Parametric_HexGrid_Generator v1 (Autodesk Fusion 360 design; units mm, degrees)
Autodesk Fusion 360 part; units mm, degrees
note: some values were not read from the file. Chosen so that the rebuilt part matches the saved one: which bodies a step acts on; which face or edge a step refers to.
sketch "Sketch1" plane through (0, 0, 0) normal (0, 1, 0) x (1, 0, 0)
  line L0 (60, 20) -> (-60, 20)
  line L1 (-60, 20) -> (-60, -20)
  line L2 (-60, -20) -> (60, -20)
  line L3 (60, -20) -> (60, 20)
  line L4 (60, 20) -> (-60, -20) construction
  line L5 (-60, 20) -> (60, -20) construction
  line L6 (-57, -17) -> (57, -17)
  line L7 (57, -17) -> (57, 17)
  line L8 (57, 17) -> (-57, 17)
  line L9 (-57, 17) -> (-57, -17)
  line L10 (6, 3.4641) -> (0, 6.9282)
  line L11 (0, 6.9282) -> (-6, 3.4641)
  line L12 (-6, 3.4641) -> (-6, -3.4641)
  line L13 (-6, -3.4641) -> (0, -6.9282)
  line L14 (0, -6.9282) -> (6, -3.4641)
  line L15 (6, -3.4641) -> (6, 3.4641)
  line L16 (0, 0) -> (3, 5.1962) construction
  line L17 (0, 0) -> (6, 0) construction
  line L18 (120, 40) -> (-120, 40)
  line L19 (-120, 40) -> (-120, -40)
  line L20 (-120, -40) -> (120, -40)
  line L21 (120, -40) -> (120, 40)
  line L22 (120, 40) -> (-120, -40) construction
  line L23 (-120, 40) -> (120, -40) construction
  dimension "d6" = 120
  dimension "d7" = 40
  dimension "d9" = 6
  dimension "d27" = 240
  dimension "d28" = 80
  constraint horizontal L0
  constraint perpendicular L0 L1
  constraint parallel L0 L2
  constraint parallel L1 L3
  constraint coincident L4 L16.start
  constraint coincident L5 L16.start
  constraint coincident L16.start L17.start
  constraint vertical L15
  constraint midpoint L10 L16.end
  constraint midpoint L15 L17.end
  constraint horizontal L18
  constraint perpendicular L18 L19
  constraint parallel L18 L20
  constraint parallel L19 L21
  constraint coincident L22 L16.start
  constraint coincident L23 L16.start
  measures "d6" distance of L1.end L2.end
  measures "d7" distance of L0.end L1.end
  measures "d9" distance of L16.start L15
  measures "d27" distance of L19.end L20.end
  measures "d28" distance of L18.end L19.end
extrude "Extrude1" add sketch "Sketch1" along normal blind 5 contours L6 L7 L8 L9 | L10 L11 L12 L13 L14 L15 makes body 1
extrude "Extrude2" cut sketch "Sketch1" along normal blind 5 contours L10 L11 L12 L13 L14 L15 bodies 1
fillet "Fillet1" radius 1 6 edges at (6, 2.5, 3.4641) (6, 2.5, -3.4641) (0, 2.5, -6.9282) (-6, 2.5, -3.4641) (-6, 2.5, 3.4641) (0, 2.5, 6.9282) on bodies 1
extrude "Extrude3" add sketch "Sketch1" along normal blind 5 contours L0 L1 L2 L3 | L18 L19 L20 L21 bodies 1
extrude "Extrude4" add sketch "Sketch1" along normal blind 5 separate body contours L0 L1 L2 L3 makes body 2
pattern_linear "R-Pattern1" count 11 spacing 15 along (1, 0, 0) both ways count 4 spacing 15 along (0.5, 0, -0.866025) both ways of "Extrude2", "Fillet1"
split "Split1" by curves path "Sketch1" along L9 L6 L7 L8 bodies 1 makes body 3 at (-109.4799, 0, 3.2539)
delete_body "RemoveBody1" bodies 3
combine "Combine1" operation add target body 2 tool bodies 1
equation "hexWidth = 12 mm"
equation "hexSpacing = 3 mm"
equation "width = 120 mm"
equation "height = 40 mm"
equation "depth = 5 mm"
equation "d6 = width"
equation "d7 = height"
equation "d8 = -hexSpacing"
equation "d9 = hexWidth / 2"
equation "d10 = depth"
equation "d12 = depth"
equation "d18 = horitzontalQTY"
equation "d19 = verticalQTY"
equation "d20 = hexWidth + hexSpacing"
equation "d21 = hexWidth + hexSpacing"
equation "d23 = depth"
equation "d25 = depth"
equation "d27 = 2 * width"
equation "d28 = 2 * height"
equation "horitzontalQTY = floor(width / hexWidth) + 1" comment "dont change"
equation "verticalQTY = floor(height / hexWidth) + 1" comment "dont change"
